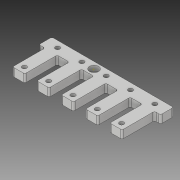
# Autodesk Inventor part: flowmeter_mount_Diego
Saved by Autodesk Inventor 2019 (Build 230136000, 136)
## iProperties
Created: 2019-12-12
Part Number: flowmeter_mount_Diego
Material: Generic
Document SubType Name: Modeling
Designer: devon
Density: 1 g/cm^3
Appearance: Default
Author: devon
Autodesk Inventor part; units mm, degrees
ref_plane "YZ Plane" through (0, 0, 0) normal (1, 0, 0) x (0, 1, 0)
ref_plane "XZ Plane" through (0, 0, 0) normal (0, 1, 0) x (-1, 0, 0)
ref_plane "XY Plane" through (0, 0, 0) normal (0, 0, 1) x (1, 0, 0)
sketch "Sketch1" plane through (0, 0, 0) normal (0, 1, 0) x (-1, 0, 0)
  line L0 (60, 8) -> (-60, 8)
  line L1 (-60, 8) -> (-60, -8)
  line L2 (-60, -8) -> (60, -8)
  line L3 (60, -8) -> (60, 8)
  line L4 (60, 8) -> (-60, -8) construction
  line L5 (-60, 8) -> (60, -8) construction
  point P0 (0, 0)
  dimension "d0" = 16
  dimension "d1" = 120
  constraints: 12 end point, 2 midpoint, 2 parallel, 1 horizontal, 1 perpendicular
  measures "d0" distance of L2.end L0.start
  measures "d1" distance of L1.end L2.end
extrude "Extrusion1" add sketch "Sketch1" along normal blind 10
hole "Hole1" at (0, 10, 0) direction (0, -1, 0) diameter 7.142 depth 25.4 counterbore diameter 11.113 counterbore depth 6.35 clearance for "Socket Head Cap Screw" size "1/4" standard "Ansi Unified Screw Threads"
sketch "Sketch2" plane through (0, 10, 0) normal (0, 1, 0) x (1, 0, 0)
  circle A0 centre (15, 0) radius 2.75
  circle A1 centre (45, 0) radius 2.75
  circle A2 centre (-15, 0) radius 2.75
  circle A3 centre (-45, 0) radius 2.75
  point P0 (0, 0)
  dimension "d15" = 5.5
  dimension "d16" = 15
  dimension "d17" = 30
  dimension "d18" = 5.5
  dimension "d19" = 15
  dimension "d20" = 5.5
  dimension "d21" = 30
  dimension "d22" = 5.5
  constraints: 4 centre point
  measures "d15" diameter of A0
  measures "d16" distance of point (0, 0) A0.centre
  measures "d17" distance of A0.centre A1.centre
  measures "d18" diameter of A1
  measures "d19" distance of point (0, 0) A2.centre
  measures "d20" diameter of A2
  measures "d21" distance of A2.centre A3.centre
  measures "d22" diameter of A3
extrude "Extrusion2" cut sketch "Sketch2" against normal up to next
sketch "Sketch4" plane through (60, 0, 8) normal (1, 0, 0) x (0, 0, -1)
  line L0 (16, 0) -> (16, 10) projected
  line L1 (0, 0) -> (0, 10) projected
  line L2 (16, 10) -> (0, 10)
  line L3 (0, 10) -> (0, 0)
  line L4 (0, 0) -> (16, 0)
  line L5 (16, 0) -> (16, 10)
  point P0 (8, 0)
  constraints: 8 end point, 2 parallel, 1 horizontal, 1 perpendicular
extrude "Extrusion3" add sketch "Sketch4" along normal blind 30
sketch "Sketch5" plane through (0, 10, 0) normal (0, 1, 0) x (1, 0, 0)
  circle A0 centre (75, 0) radius 2.75
  circle A1 centre (45, 0) radius 2.75 projected
  point P0 (0, 0)
  dimension "d29" = 5.5
  dimension "d30" = 30
  constraints: 1 centre point
  measures "d29" diameter of A0
  measures "d30" distance of A1.centre A0.centre
extrude "Extrusion4" cut sketch "Sketch5" against normal up to next contours A0
sketch "Sketch6" plane through (-60, 0, 8) normal (0, 0, 1) x (1, 0, 0)
  line L0 (0, 10) -> (150, 10) projected
  line L1 (0, 0) -> (150, 0) projected
  line L2 (7.5, 10) -> (22.5, 10)
  line L3 (22.5, 10) -> (22.5, 0)
  line L4 (22.5, 0) -> (7.5, 0)
  line L5 (7.5, 0) -> (7.5, 10)
  line L6 (0, 0) -> (0, 10) projected
  line L7 (0, 10) -> (150, 10) projected
  line L8 (37.5, 10) -> (52.5, 10)
  line L9 (52.5, 10) -> (52.5, 0)
  line L10 (52.5, 0) -> (37.5, 0)
  line L11 (37.5, 0) -> (37.5, 10)
  line L12 (67.5, 10) -> (82.5, 10)
  line L13 (82.5, 10) -> (82.5, 0)
  line L14 (82.5, 0) -> (67.5, 0)
  line L15 (67.5, 0) -> (67.5, 10)
  line L16 (97.5, 10) -> (112.5, 10)
  line L17 (112.5, 10) -> (112.5, 0)
  line L18 (112.5, 0) -> (97.5, 0)
  line L19 (97.5, 0) -> (97.5, 10)
  line L20 (127.5, 10) -> (142.5, 10)
  line L21 (142.5, 10) -> (142.5, 0)
  line L22 (142.5, 0) -> (127.5, 0)
  line L23 (127.5, 0) -> (127.5, 10)
  point P0 (60, 0)
  dimension "d33" = 15
  dimension "d34" = 7.5
  dimension "d35" = 15
  dimension "d36" = 15
  dimension "d37" = 15
  dimension "d38" = 15
  dimension "d39" = 15
  dimension "d40" = 15
  dimension "d41" = 15
  dimension "d42" = 15
  constraints: 40 end point, 10 parallel, 10 point on line, 5 horizontal, 5 perpendicular
  measures "d33" distance between parallel lines of L3 L5
  measures "d34" distance between parallel lines of L6 L5
  measures "d35" distance between parallel lines of L11 L9
  measures "d36" distance between parallel lines of L3 L11
  measures "d37" distance between parallel lines of L13 L15
  measures "d38" distance between parallel lines of L17 L19
  measures "d39" distance between parallel lines of L21 L23
  measures "d40" distance between parallel lines of L15 L9
  measures "d41" distance between parallel lines of L19 L13
  measures "d42" distance between parallel lines of L23 L17
extrude "Extrusion5" add sketch "Sketch6" along normal blind 40 contours L0 L3 L1 L5 | L0 L9 L1 L11 | L0 L13 L1 L15 | L0 L17 L1 L19 | L0 L21 L1 L23
sketch "Sketch7" plane through (0, 10, 0) normal (0, 1, 0) x (1, 0, 0)
  circle A0 centre (-45, -41) radius 2.75
  circle A1 centre (-45, 0) radius 2.75 projected
  line L0 (-52.5, -8) -> (-52.5, -48) projected
  circle A2 centre (-15, -41) radius 2.75
  circle A3 centre (15, -41) radius 2.75
  circle A4 centre (45, -41) radius 2.75
  circle A5 centre (75, -41) radius 2.75
  point P0 (0, 0)
  dimension "d45" = 5.5
  dimension "d46" = 41
  dimension "d47" = 7.5
  dimension "d48" = 5.5
  dimension "d49" = 5.5
  dimension "d50" = 5.5
  dimension "d51" = 5.5
  constraints: 5 centre point
  measures "d45" diameter of A0
  measures "d46" distance of A1.centre A0.centre
  measures "d47" distance from line of L0 A0.centre
  measures "d48" diameter of A2
  measures "d49" diameter of A3
  measures "d50" diameter of A4
  measures "d51" diameter of A5
extrude "Extrusion6" cut sketch "Sketch7" against normal up to next contours A0 | A2 | A3 | A4 | A5
fillet "Fillet1" radius 2 24 edges at (-52.5, 5, 48) (-37.5, 5, 48) (-22.5, 5, 48) (-7.5, 5, 48) (7.5, 5, 48) (22.5, 5, 48) (37.5, 5, 48) (52.5, 5, 48) (67.5, 5, 48) (82.5, 5, 48) (90, 5, 8) (90, 5, -8) (-60, 5, 8) (-60, 5, -8) (-52.5, 5, 8) (-37.5, 5, 8) (-22.5, 5, 8) (7.5, 5, 8) (37.5, 5, 8) (67.5, 5, 8) (82.5, 5, 8) (52.5, 5, 8) (22.5, 5, 8) (-7.5, 5, 8)
body "Solid1"
